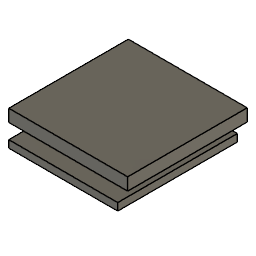
ASFALT_LINE_FOLLOWER_MOTOR_MOUNT_V0 (Autodesk Fusion 360 design; units mm, degrees)
Autodesk Fusion 360 part; units mm, degrees
sketch "Sketch1" plane through (0, 0, 0) normal (0, 0, 1) x (1, 0, 0)
  line L0 (8.375, 6.75) -> (-8.375, 6.75)
  line L1 (-8.375, -6.75) -> (8.375, -6.75)
  line L2 (8.375, -6.75) -> (8.375, 6.75)
  line L3 (8.375, 6.75) -> (-8.375, -6.75) construction
  line L4 (-8.375, 6.75) -> (8.375, -6.75) construction
  line L5 (-9, 12.0754) -> (13, 12.0754)
  line L6 (13, 12.0754) -> (13, -12.0754)
  line L7 (13, -12.0754) -> (-9, -12.0754)
  line L8 (-9, -12.0754) -> (-9, 12.0754)
  line L9 (-9, 12.0754) -> (13, -12.0754) construction
  line L10 (13, 12.0754) -> (-9, -12.0754) construction
  line L11 (-8.375, -6.75) -> (-9, -6.75)
  line L12 (-8.375, 6.75) -> (-9, 6.75)
  point P0 (2, 0)
  dimension "d1" = 16.75
  dimension "d2" = 13.5
  constraint horizontal L0
  constraint parallel L0 L1
  constraint coincident L3 origin
  constraint coincident L4 origin
  constraint horizontal L5
  constraint perpendicular L5 L6
  constraint parallel L5 L7
  constraint parallel L6 L8
  constraint coincident L9 P0
  constraint coincident L10 P0
  constraint coincident L8 L11.end
  constraint perpendicular L8 L11
  constraint coincident L8 L12.end
  constraint perpendicular L8 L12
  measures "d1" distance of L1.start L1.end
  measures "d2" distance of L0.end L1.start
extrude "Extrude1" add sketch "Sketch1" along normal blind 7
extrude "Extrude2" cut sketch "Sketch1" along normal blind 4.5 and the other way blind -1.5 contours L0 L1 L2 L5 L6 L7 L8 L11 L12
extrude "Extrude3" add 1 faces at (13, 4.0251, 6.1667) along direction (1, 0, 0) blind 2
